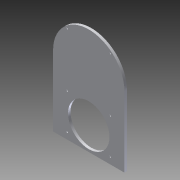
# Autodesk Inventor part: Bottom_Deck
Saved by Autodesk Inventor 2011 SP1 (Build 150282100, 282)
## iProperties
Created: 2011-06-12
Part Number: Bottom_Deck
Document SubType Name: Modeling
Designer: Andrew G. Meyer
Mass: 790.425 g
Surface Area: 1836.86 cm^2
Volume: 790.425 cm^3
Density: 1 g/cm^3
Author: Andrew G. Meyer
Autodesk Inventor part; units mm, degrees
ref_plane "YZ Plane" through (0, 0, 0) normal (1, 0, 0) x (0, 1, 0)
ref_plane "XZ Plane" through (0, 0, 0) normal (0, 1, 0) x (-1, 0, 0)
ref_plane "XY Plane" through (0, 0, 0) normal (0, 0, 1) x (1, 0, 0)
sketch "Sketch1" plane through (0, 0, 0) normal (0, 0, 1) x (1, 0, 0)
  line L0 (-136.525, 0) -> (-136.525, -269.875)
  line L1 (-136.525, -269.875) -> (136.525, -269.875)
  line L2 (136.525, -269.875) -> (136.525, 0)
  arc A0 (136.525, 0) -> (-136.525, 0) centre (0, 0) ccw
  dimension "d0" = 273.05
  dimension "d1" = 406.4
  constraints: 6 end point, 2 point on circle, 2 tangent, 1 centre point, 1 coincident, 1 parallel, 1 perpendicular, 1 vertical
  measures "d0" distance of L0.end L1.end
extrude "Extrusion1" add sketch "Sketch1" along normal blind 9.525
hole "Hole1" at (-82.55, -244.475, 9.525) direction (0, 0, -1) diameter 6.35 depth 25.4 tip angle 118
hole "Hole2" at (82.55, -244.475, 9.525) direction (0, 0, -1) diameter 6.35 depth 25.4 tip angle 118
hole "Hole3" at (-82.55, -107.95, 9.525) direction (0, 0, -1) diameter 6.35 depth 25.4 tip angle 118
hole "Hole4" at (82.55, -107.95, 9.525) direction (0, 0, -1) diameter 6.35 depth 25.4 tip angle 118
hole "Hole5" at (-82.55, 98.425, 9.525) direction (0, 0, -1) diameter 6.35 depth 25.4 tip angle 118
hole "Hole6" at (82.55, 98.425, 9.525) direction (0, 0, -1) diameter 6.35 depth 25.4 tip angle 118
hole "Hole7" at (0, -180.975, 9.525) direction (0, 0, -1) diameter 158.75 depth 25.4 tip angle 118
body "Solid1"
